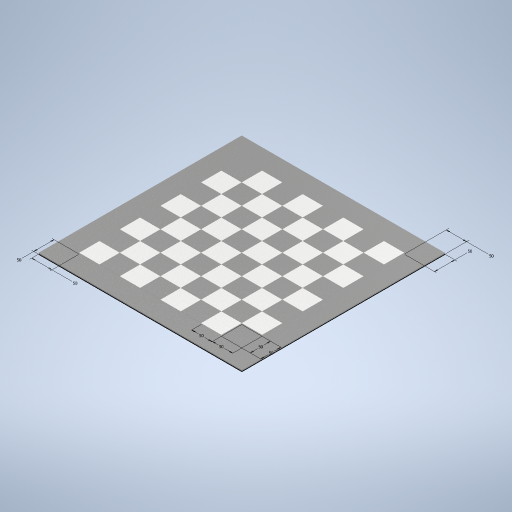
# Autodesk Inventor part: Board
Saved by Autodesk Inventor 2024 (Build 280153000, 153)
## iProperties
Created: 2023-07-19
Part Number: Board
Material: Generic
Document SubType Name: Modeling
Designer: Bruno
Density: 1 g/cm^3
Appearance: Black Tile Material
Author: Bruno
Autodesk Inventor part; units mm, degrees
ref_plane "YZ Plane" through (0, 0, 0) normal (1, 0, 0) x (0, 1, 0)
ref_plane "XZ Plane" through (0, 0, 0) normal (0, 1, 0) x (-1, 0, 0)
ref_plane "XY Plane" through (0, 0, 0) normal (0, 0, 1) x (1, 0, 0)
sketch "Sketch1" plane through (0, 0, 0) normal (0, 1, 0) x (-1, 0, 0)
  line L0 (50, 0) -> (0, 0)
  line L1 (0, 0) -> (0, -50)
  line L2 (0, -50) -> (50, -50)
  line L3 (50, -50) -> (50, 0)
  line L4 (100, 0) -> (50, 0)
  line L5 (50, 0) -> (50, -50)
  line L6 (50, -50) -> (100, -50)
  line L7 (100, -50) -> (100, 0)
  line L8 (150, 0) -> (100, 0)
  line L9 (100, 0) -> (100, -50)
  line L10 (100, -50) -> (150, -50)
  line L11 (150, -50) -> (150, 0)
  line L12 (200, 0) -> (150, 0)
  line L13 (150, 0) -> (150, -50)
  line L14 (150, -50) -> (200, -50)
  line L15 (200, -50) -> (200, 0)
  line L16 (250, 0) -> (200, 0)
  line L17 (200, 0) -> (200, -50)
  line L18 (200, -50) -> (250, -50)
  line L19 (250, -50) -> (250, 0)
  line L20 (300, 0) -> (250, 0)
  line L21 (250, 0) -> (250, -50)
  line L22 (250, -50) -> (300, -50)
  line L23 (300, -50) -> (300, 0)
  line L24 (350, 0) -> (300, 0)
  line L25 (300, 0) -> (300, -50)
  line L26 (300, -50) -> (350, -50)
  line L27 (350, -50) -> (350, 0)
  line L28 (400, 0) -> (350, 0)
  line L29 (350, 0) -> (350, -50)
  line L30 (350, -50) -> (400, -50)
  line L31 (400, -50) -> (400, 0)
  line L32 (50, -50) -> (0, -50)
  line L33 (0, -50) -> (0, -100)
  line L34 (0, -100) -> (50, -100)
  line L35 (50, -100) -> (50, -50)
  line L36 (100, -50) -> (50, -50)
  line L37 (50, -50) -> (50, -100)
  line L38 (50, -100) -> (100, -100)
  line L39 (100, -100) -> (100, -50)
  line L40 (150, -50) -> (100, -50)
  line L41 (100, -50) -> (100, -100)
  line L42 (100, -100) -> (150, -100)
  line L43 (150, -100) -> (150, -50)
  line L44 (200, -50) -> (150, -50)
  line L45 (150, -50) -> (150, -100)
  line L46 (150, -100) -> (200, -100)
  line L47 (200, -100) -> (200, -50)
  line L48 (250, -50) -> (200, -50)
  line L49 (200, -50) -> (200, -100)
  line L50 (200, -100) -> (250, -100)
  line L51 (250, -100) -> (250, -50)
  line L52 (300, -50) -> (250, -50)
  line L53 (250, -50) -> (250, -100)
  line L54 (250, -100) -> (300, -100)
  line L55 (300, -100) -> (300, -50)
  line L56 (350, -50) -> (300, -50)
  line L57 (300, -50) -> (300, -100)
  line L58 (300, -100) -> (350, -100)
  line L59 (350, -100) -> (350, -50)
  line L60 (400, -50) -> (350, -50)
  line L61 (350, -50) -> (350, -100)
  line L62 (350, -100) -> (400, -100)
  line L63 (400, -100) -> (400, -50)
  line L64 (50, -100) -> (0, -100)
  line L65 (0, -100) -> (0, -150)
  line L66 (0, -150) -> (50, -150)
  line L67 (50, -150) -> (50, -100)
  line L68 (100, -100) -> (50, -100)
  line L69 (50, -100) -> (50, -150)
  line L70 (50, -150) -> (100, -150)
  line L71 (100, -150) -> (100, -100)
  line L72 (150, -100) -> (100, -100)
  line L73 (100, -100) -> (100, -150)
  line L74 (100, -150) -> (150, -150)
  line L75 (150, -150) -> (150, -100)
  line L76 (200, -100) -> (150, -100)
  line L77 (150, -100) -> (150, -150)
  line L78 (150, -150) -> (200, -150)
  line L79 (200, -150) -> (200, -100)
  line L80 (250, -100) -> (200, -100)
  line L81 (200, -100) -> (200, -150)
  line L82 (200, -150) -> (250, -150)
  line L83 (250, -150) -> (250, -100)
  line L84 (300, -100) -> (250, -100)
  line L85 (250, -100) -> (250, -150)
  line L86 (250, -150) -> (300, -150)
  line L87 (300, -150) -> (300, -100)
  line L88 (350, -100) -> (300, -100)
  line L89 (300, -100) -> (300, -150)
  line L90 (300, -150) -> (350, -150)
  line L91 (350, -150) -> (350, -100)
  line L92 (400, -100) -> (350, -100)
  line L93 (350, -100) -> (350, -150)
  line L94 (350, -150) -> (400, -150)
  line L95 (400, -150) -> (400, -100)
  line L96 (50, -150) -> (0, -150)
  line L97 (0, -150) -> (0, -200)
  line L98 (0, -200) -> (50, -200)
  line L99 (50, -200) -> (50, -150)
  line L100 (100, -150) -> (50, -150)
  line L101 (50, -150) -> (50, -200)
  line L102 (50, -200) -> (100, -200)
  line L103 (100, -200) -> (100, -150)
  line L104 (150, -150) -> (100, -150)
  line L105 (100, -150) -> (100, -200)
  line L106 (100, -200) -> (150, -200)
  line L107 (150, -200) -> (150, -150)
  line L108 (200, -150) -> (150, -150)
  line L109 (150, -150) -> (150, -200)
  line L110 (150, -200) -> (200, -200)
  line L111 (200, -200) -> (200, -150)
  line L112 (250, -150) -> (200, -150)
  line L113 (200, -150) -> (200, -200)
  line L114 (200, -200) -> (250, -200)
  line L115 (250, -200) -> (250, -150)
  line L116 (300, -150) -> (250, -150)
  line L117 (250, -150) -> (250, -200)
  line L118 (250, -200) -> (300, -200)
  line L119 (300, -200) -> (300, -150)
  line L120 (350, -150) -> (300, -150)
  line L121 (300, -150) -> (300, -200)
  line L122 (300, -200) -> (350, -200)
  line L123 (350, -200) -> (350, -150)
  line L124 (400, -150) -> (350, -150)
  line L125 (350, -150) -> (350, -200)
  line L126 (350, -200) -> (400, -200)
  line L127 (400, -200) -> (400, -150)
  line L128 (50, -200) -> (0, -200)
  line L129 (0, -200) -> (0, -250)
  line L130 (0, -250) -> (50, -250)
  line L131 (50, -250) -> (50, -200)
  line L132 (100, -200) -> (50, -200)
  line L133 (50, -200) -> (50, -250)
  line L134 (50, -250) -> (100, -250)
  line L135 (100, -250) -> (100, -200)
  line L136 (150, -200) -> (100, -200)
  line L137 (100, -200) -> (100, -250)
  line L138 (100, -250) -> (150, -250)
  line L139 (150, -250) -> (150, -200)
  line L140 (200, -200) -> (150, -200)
  line L141 (150, -200) -> (150, -250)
  line L142 (150, -250) -> (200, -250)
  line L143 (200, -250) -> (200, -200)
  line L144 (250, -200) -> (200, -200)
  line L145 (200, -200) -> (200, -250)
  line L146 (200, -250) -> (250, -250)
  line L147 (250, -250) -> (250, -200)
  line L148 (300, -200) -> (250, -200)
  line L149 (250, -200) -> (250, -250)
  line L150 (250, -250) -> (300, -250)
  line L151 (300, -250) -> (300, -200)
  line L152 (350, -200) -> (300, -200)
  line L153 (300, -200) -> (300, -250)
  line L154 (300, -250) -> (350, -250)
  line L155 (350, -250) -> (350, -200)
  line L156 (400, -200) -> (350, -200)
  line L157 (350, -200) -> (350, -250)
  line L158 (350, -250) -> (400, -250)
  line L159 (400, -250) -> (400, -200)
  line L160 (50, -250) -> (0, -250)
  line L161 (0, -250) -> (0, -300)
  line L162 (0, -300) -> (50, -300)
  line L163 (50, -300) -> (50, -250)
  line L164 (100, -250) -> (50, -250)
  line L165 (50, -250) -> (50, -300)
  line L166 (50, -300) -> (100, -300)
  line L167 (100, -300) -> (100, -250)
  line L168 (150, -250) -> (100, -250)
  line L169 (100, -250) -> (100, -300)
  line L170 (100, -300) -> (150, -300)
  line L171 (150, -300) -> (150, -250)
  line L172 (200, -250) -> (150, -250)
  line L173 (150, -250) -> (150, -300)
  line L174 (150, -300) -> (200, -300)
  line L175 (200, -300) -> (200, -250)
  line L176 (250, -250) -> (200, -250)
  line L177 (200, -250) -> (200, -300)
  line L178 (200, -300) -> (250, -300)
  line L179 (250, -300) -> (250, -250)
  line L180 (300, -250) -> (250, -250)
  line L181 (250, -250) -> (250, -300)
  line L182 (250, -300) -> (300, -300)
  line L183 (300, -300) -> (300, -250)
  line L184 (350, -250) -> (300, -250)
  line L185 (300, -250) -> (300, -300)
  line L186 (300, -300) -> (350, -300)
  line L187 (350, -300) -> (350, -250)
  line L188 (400, -250) -> (350, -250)
  line L189 (350, -250) -> (350, -300)
  line L190 (350, -300) -> (400, -300)
  line L191 (400, -300) -> (400, -250)
  line L192 (50, -300) -> (0, -300)
  line L193 (0, -300) -> (0, -350)
  line L194 (0, -350) -> (50, -350)
  line L195 (50, -350) -> (50, -300)
  line L196 (100, -300) -> (50, -300)
  line L197 (50, -300) -> (50, -350)
  line L198 (50, -350) -> (100, -350)
  line L199 (100, -350) -> (100, -300)
  line L200 (150, -300) -> (100, -300)
  line L201 (100, -300) -> (100, -350)
  line L202 (100, -350) -> (150, -350)
  line L203 (150, -350) -> (150, -300)
  line L204 (200, -300) -> (150, -300)
  line L205 (150, -300) -> (150, -350)
  line L206 (150, -350) -> (200, -350)
  line L207 (200, -350) -> (200, -300)
  line L208 (250, -300) -> (200, -300)
  line L209 (200, -300) -> (200, -350)
  line L210 (200, -350) -> (250, -350)
  line L211 (250, -350) -> (250, -300)
  line L212 (300, -300) -> (250, -300)
  line L213 (250, -300) -> (250, -350)
  line L214 (250, -350) -> (300, -350)
  line L215 (300, -350) -> (300, -300)
  line L216 (350, -300) -> (300, -300)
  line L217 (300, -300) -> (300, -350)
  line L218 (300, -350) -> (350, -350)
  line L219 (350, -350) -> (350, -300)
  line L220 (400, -300) -> (350, -300)
  line L221 (350, -300) -> (350, -350)
  line L222 (350, -350) -> (400, -350)
  line L223 (400, -350) -> (400, -300)
  line L224 (50, -350) -> (0, -350)
  line L225 (0, -350) -> (0, -400)
  line L226 (0, -400) -> (50, -400)
  line L227 (50, -400) -> (50, -350)
  line L228 (100, -350) -> (50, -350)
  line L229 (50, -350) -> (50, -400)
  line L230 (50, -400) -> (100, -400)
  line L231 (100, -400) -> (100, -350)
  line L232 (150, -350) -> (100, -350)
  line L233 (100, -350) -> (100, -400)
  line L234 (100, -400) -> (150, -400)
  line L235 (150, -400) -> (150, -350)
  line L236 (200, -350) -> (150, -350)
  line L237 (150, -350) -> (150, -400)
  line L238 (150, -400) -> (200, -400)
  line L239 (200, -400) -> (200, -350)
  line L240 (250, -350) -> (200, -350)
  line L241 (200, -350) -> (200, -400)
  line L242 (200, -400) -> (250, -400)
  line L243 (250, -400) -> (250, -350)
  line L244 (300, -350) -> (250, -350)
  line L245 (250, -350) -> (250, -400)
  line L246 (250, -400) -> (300, -400)
  line L247 (300, -400) -> (300, -350)
  line L248 (350, -350) -> (300, -350)
  line L249 (300, -350) -> (300, -400)
  line L250 (300, -400) -> (350, -400)
  line L251 (350, -400) -> (350, -350)
  line L252 (400, -350) -> (350, -350)
  line L253 (350, -350) -> (350, -400)
  line L254 (350, -400) -> (400, -400)
  line L255 (400, -400) -> (400, -350)
  line L256 (-50, 50) -> (450, 50)
  line L257 (450, 50) -> (450, -450)
  line L258 (450, -450) -> (-50, -450)
  line L259 (-50, -450) -> (-50, 50)
  point P0 (50, -50)
  point P1 (50, -50)
  point P2 (50, -50)
  point P3 (50, -50)
  point P4 (50, -50)
  point P5 (350, 0)
  point P6 (250, 0)
  point P7 (150, 0)
  point P8 (50, 0)
  point P9 (300, 0)
  point P10 (200, 0)
  point P11 (100, 0)
  point P12 (50, 0)
  point P13 (100, 0)
  point P14 (150, 0)
  point P15 (200, 0)
  point P16 (250, 0)
  point P17 (300, 0)
  point P18 (350, 0)
  dimension "d0" = 50
  dimension "d1" = 50
  dimension "d4" = 50
  dimension "d7" = 50
  dimension "d10" = 50
  dimension "d12" = 50
  dimension "d13" = 50
  dimension "d14" = 50
  constraints: 520 end point, 4 parallel, 3 horizontal, 2 collinear, 2 perpendicular, 1 coincident, 1 vertical, 502 other
  measures "d0" distance between parallel lines of L1 L3
  measures "d1" distance of L2.end L0.start
  measures "d4" distance of L0.start L4.start
  measures "d7" distance of L0.start L32.start
  measures "d10" distance between parallel lines of L258 L226
  measures "d12" distance between parallel lines of L28 L256
  measures "d13" distance between parallel lines of L257 L31
  measures "d14" distance between parallel lines of L225 L259
extrude "WhiteTiles" add sketch "Sketch1" along normal blind 3.1 contours L3 L2 L1 L0 | L6 L39 L38 L35 | L8 L11 L10 L7 | L67 L66 L65 L34 | L14 L47 L46 L43 | L42 L75 L74 L71 | L70 L103 L102 L99 | L16 L19 L18 L15 | L131 L130 L129 L98 | L22 L55 L54 L51 | L50 L83 L82 L79 | L78 L111 L110 L107 | L106 L139 L138 L135 | L134 L167 L166 L163 | L24 L27 L26 L23 | L195 L194 L193 L162 | L30 L63 L62 L59 | L58 L91 L90 L87 | L86 L119 L118 L115 | L114 L147 L146 L143 | L142 L175 L174 L171 | L170 L203 L202 L199 | L198 L231 L230 L227 | L94 L127 L126 L123 | L122 L155 L154 L151 | L150 L183 L182 L179 | L178 L211 L210 L207 | L206 L239 L238 L235 | L158 L191 L190 L187 | L186 L219 L218 L215 | L214 L247 L246 L243 | L222 L255 L254 L251
extrude "BlackTiles" add sketch "Sketch1" along normal blind 3 contours L4 L7 L6 L3 | L35 L34 L33 L2 | L10 L43 L42 L39 | L38 L71 L70 L67 | L12 L15 L14 L11 | L99 L98 L97 L66 | L18 L51 L50 L47 | L46 L79 L78 L75 | L74 L107 L106 L103 | L102 L135 L134 L131 | L20 L23 L22 L19 | L163 L162 L161 L130 | L26 L59 L58 L55 | L54 L87 L86 L83 | L82 L115 L114 L111 | L110 L143 L142 L139 | L138 L171 L170 L167 | L166 L199 L198 L195 | L28 L31 L30 L27 | L227 L226 L225 L194 | L62 L95 L94 L91 | L90 L123 L122 L119 | L118 L151 L150 L147 | L146 L179 L178 L175 | L174 L207 L206 L203 | L202 L235 L234 L231 | L126 L159 L158 L155 | L154 L187 L186 L183 | L182 L215 L214 L211 | L210 L243 L242 L239 | L190 L223 L222 L219 | L218 L251 L250 L247
extrude "Extrusion3" add sketch "Sketch1" along normal blind 2.9
body "Solid1"
